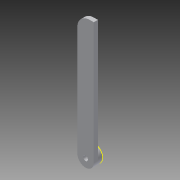
# Autodesk Inventor part: PinewoodStartArm
Saved by Autodesk Inventor 2013 (Build 170138000, 138)
## iProperties
Created: 2015-05-14
Part Number: PinewoodStartArm
Material: Generic
Document SubType Name: Modeling
Designer: joshgunnar
Density: 1 g/cm^3
Author: joshgunnar
Autodesk Inventor part; units mm, degrees
ref_plane "YZ Plane" through (0, 0, 0) normal (1, 0, 0) x (0, 1, 0)
ref_plane "XZ Plane" through (0, 0, 0) normal (0, 1, 0) x (-1, 0, 0)
ref_plane "XY Plane" through (0, 0, 0) normal (0, 0, 1) x (1, 0, 0)
sketch "Sketch1" plane through (0, 0, 0) normal (0, 0, 1) x (1, 0, 0)
  circle A0 centre (0, 0) radius 6
  line L0 (-6, 0) -> (6, 0)
  line L1 (6, 0) -> (6, 88.9)
  line L2 (6, 88.9) -> (-6, 88.9)
  line L3 (-6, 88.9) -> (-6, 0)
  dimension "d0" = 12
  dimension "d1" = 88.9
  constraints: 8 end point, 2 parallel, 1 coincident, 1 horizontal, 1 horizontal alignment, 1 perpendicular, 2 other
  measures "d1" distance of L1.end L0.end
extrude "Extrusion1" add sketch "Sketch1" along normal blind 3
sketch "Sketch2" plane through (0, 0, 0) normal (0, 0, -1) x (-1, 0, 0)
  arc A0 (-6, 0) -> (6, 0) centre (0, 0) ccw projected
  circle A1 centre (0, 0) radius 6
  dimension "d4" = 12
  constraints: 1 centre point, 1 coincident
  measures "d4" diameter of A1
extrude "Extrusion2" add sketch "Sketch2" along normal blind 3.5
sketch "Sketch3" plane through (0, 0, -3.5) normal (0, 0, -1) x (-1, 0, 0)
  circle A0 centre (0, 0) radius 6 projected
  circle A1 centre (0, 0) radius 2.9
  dimension "d7" = 5.8
  constraints: 1 centre point, 1 coincident
  measures "d7" diameter of A1
extrude "Extrusion3" cut sketch "Sketch3" against normal blind 3.5 contours A1
sketch "Sketch5" plane through (0, 0, 0) normal (0, 0, -1) x (-1, 0, 0)
  line L0 (-2.998, 23.4218) -> (-2.998, 33.3533) construction
  line L1 (-2.998, 33.3533) -> (56.8825, 33.3533) construction
  line L2 (56.8825, 33.3533) -> (56.8825, 23.4218) construction
  line L3 (56.8825, 23.4218) -> (-2.998, 23.4218) construction
  spline S0 degree 2 poles (3.3195, 27.1936) (3.3195, 26.1456) (3.0476, 24.5538) (2.8499, 23.8717) knots 0 0 0 1 2 2 2
  line L4 (2.8499, 23.8717) -> (1.3966, 23.8717)
  line L5 (1.3966, 23.8717) -> (1.3966, 24.0793)
  spline S1 degree 2 poles (1.3966, 24.0793) (1.7871, 24.7664) (2.2073, 26.4273) (2.2073, 27.2084) knots 0 0 0 1 2 2 2
  spline S2 degree 2 poles (2.2073, 27.2084) (2.2073, 27.4012) (2.148, 28.0487) (2.0886, 28.2415) knots 0 0 0 1 2 2 2
  spline S3 degree 2 poles (2.0886, 28.2415) (2.0194, 28.4838) (1.7673, 28.8149) (1.5647, 28.8149) knots 0 0 0 1 2 2 2
  spline S4 degree 2 poles (1.5647, 28.8149) (1.3323, 28.8149) (1.0456, 28.2761) (0.9814, 27.9004) knots 0 0 0 1 2 2 2
  spline S5 degree 2 poles (0.9814, 27.9004) (0.8973, 27.4308) (0.754, 26.373) (0.6452, 25.9083) knots 0 0 0 1 2 2 2
  spline S6 degree 2 poles (0.6452, 25.9083) (0.398, 24.8455) (-0.4473, 23.9261) (-1.08, 23.9261) knots 0 0 0 1 2 2 2
  spline S7 degree 2 poles (-1.08, 23.9261) (-1.9352, 23.9261) (-2.998, 26.1011) (-2.998, 27.7274) knots 0 0 0 1 2 2 2
  spline S8 degree 2 poles (-2.998, 27.7274) (-2.998, 28.548) (-2.7755, 30.1645) (-2.5877, 30.8021) knots 0 0 0 1 2 2 2
  line L6 (-2.5877, 30.8021) -> (-1.1937, 30.8021)
  line L7 (-1.1937, 30.8021) -> (-1.1937, 30.5995)
  spline S9 degree 2 poles (-1.1937, 30.5995) (-1.4853, 30.0903) (-1.8857, 28.6222) (-1.8857, 27.8461) knots 0 0 0 1 2 2 2
  spline S10 degree 2 poles (-1.8857, 27.8461) (-1.8857, 27.5445) (-1.8264, 27.065) (-1.7473, 26.803) knots 0 0 0 1 2 2 2
  spline S11 degree 2 poles (-1.7473, 26.803) (-1.6831, 26.5855) (-1.426, 26.2741) (-1.2678, 26.2741) knots 0 0 0 1 2 2 2
  spline S12 degree 2 poles (-1.2678, 26.2741) (-1.0306, 26.2741) (-0.7587, 26.7734) (-0.6499, 27.4852) knots 0 0 0 1 2 2 2
  spline S13 degree 2 poles (-0.6499, 27.4852) (-0.5807, 27.9449) (-0.4473, 28.8001) (-0.3336, 29.2846) knots 0 0 0 1 2 2 2
  spline S14 degree 2 poles (-0.3336, 29.2846) (-0.1012, 30.2337) (0.6699, 31.163) (1.3027, 31.163) knots 0 0 0 1 2 2 2
  spline S15 degree 2 poles (1.3027, 31.163) (2.2122, 31.163) (3.3195, 29.0176) (3.3195, 27.1936) knots 0 0 0 1 2 2 2
  line L8 (3.2108, 34.0894) -> (-1.7276, 34.0894)
  line L9 (-1.7276, 34.0894) -> (-1.7276, 31.3855)
  line L10 (-1.7276, 31.3855) -> (-2.8892, 31.3855)
  line L11 (-2.8892, 31.3855) -> (-2.8892, 39.092)
  line L12 (-2.8892, 39.092) -> (-1.7276, 39.092)
  line L13 (-1.7276, 39.092) -> (-1.7276, 36.388)
  line L14 (-1.7276, 36.388) -> (3.2108, 36.388)
  line L15 (3.2108, 36.388) -> (3.2108, 34.0894)
  line L16 (3.2108, 39.0525) -> (-2.8892, 42.142)
  line L17 (-2.8892, 42.142) -> (-2.8892, 44.6433)
  line L18 (-2.8892, 44.6433) -> (3.2108, 47.7329)
  line L19 (3.2108, 47.7329) -> (3.2108, 45.365)
  line L20 (3.2108, 45.365) -> (1.9651, 44.7966)
  line L21 (1.9651, 44.7966) -> (1.9651, 41.9295)
  line L22 (1.9651, 41.9295) -> (3.2108, 41.356)
  line L23 (3.2108, 41.356) -> (3.2108, 39.0525)
  line L24 (0.8578, 44.2923) -> (-1.1492, 43.363)
  line L25 (-1.1492, 43.363) -> (0.8578, 42.4337)
  line L26 (0.8578, 42.4337) -> (0.8578, 44.2923)
  line L27 (3.2108, 57.1053) -> (3.2108, 54.3074)
  line L28 (3.2108, 54.3074) -> (0.9715, 51.7567)
  line L29 (0.9715, 51.7567) -> (0.9715, 50.9262)
  line L30 (0.9715, 50.9262) -> (3.2108, 50.9262)
  line L31 (3.2108, 50.9262) -> (3.2108, 48.6424)
  line L32 (3.2108, 48.6424) -> (-2.8892, 48.6424)
  line L33 (-2.8892, 48.6424) -> (-2.8892, 52.3252)
  spline S16 degree 2 poles (-2.8892, 52.3252) (-2.8892, 53.0864) (-2.7607, 54.2184) (-2.563, 54.6979) knots 0 0 0 1 2 2 2
  spline S17 degree 2 poles (-2.563, 54.6979) (-2.3554, 55.1873) (-1.7078, 55.7657) (-1.2135, 55.7657) knots 0 0 0 1 2 2 2
  spline S18 degree 2 poles (-1.2135, 55.7657) (-0.5165, 55.7657) (0.3585, 54.8215) (0.6155, 54.0256) knots 0 0 0 1 2 2 2
  line L34 (0.6155, 54.0256) -> (3.2108, 57.1053)
  spline S19 degree 2 poles (-1.0207, 53.4077) (-1.253, 53.4077) (-1.5842, 53.1408) (-1.6732, 52.8343) knots 0 0 0 1 2 2 2
  spline S20 degree 2 poles (-1.6732, 52.8343) (-1.7325, 52.6218) (-1.7671, 52.0879) (-1.7671, 51.6974) knots 0 0 0 1 2 2 2
  line L35 (-1.7671, 51.6974) -> (-1.7671, 50.9262)
  line L36 (-1.7671, 50.9262) -> (-0.1259, 50.9262)
  line L37 (-0.1259, 50.9262) -> (-0.1259, 51.5837)
  spline S21 degree 2 poles (-0.1259, 51.5837) (-0.1259, 52.0632) (-0.205, 52.7355) (-0.3286, 52.9727) knots 0 0 0 1 2 2 2
  spline S22 degree 2 poles (-0.3286, 52.9727) (-0.4473, 53.1902) (-0.7636, 53.4077) (-1.0207, 53.4077) knots 0 0 0 1 2 2 2
  line L38 (3.2108, 59.5374) -> (-1.7276, 59.5374)
  line L39 (-1.7276, 59.5374) -> (-1.7276, 56.8334)
  line L40 (-1.7276, 56.8334) -> (-2.8892, 56.8334)
  line L41 (-2.8892, 56.8334) -> (-2.8892, 64.54)
  line L42 (-2.8892, 64.54) -> (-1.7276, 64.54)
  line L43 (-1.7276, 64.54) -> (-1.7276, 61.836)
  line L44 (-1.7276, 61.836) -> (3.2108, 61.836)
  line L45 (3.2108, 61.836) -> (3.2108, 59.5374)
  constraints: 2 other
extrude "Extrusion5" add sketch "Sketch5" along normal blind 1.5
sketch "Sketch6" plane through (0, 0, 3) normal (0, 0, 1) x (1, 0, 0)
  arc A0 (-6, 0) -> (6, 0) centre (0, 0) ccw projected
  circle A1 centre (0, 0) radius 1.75
  dimension "d18" = 3.5
  constraints: 1 centre point, 1 coincident
  measures "d18" diameter of A1
extrude "Extrusion6" cut sketch "Sketch6" against normal through all
fillet "Fillet2" radius 9 1 edges at (-6, 88.9, 1.5)
sketch "Sketch7" plane through (0, 0, -3.5) normal (0, 0, -1) x (-1, 0, 0)
  circle A0 centre (0, 0) radius 2.9 projected
  circle A1 centre (0, 0) radius 6 projected
sketch "Sketch8" plane through (0, 0, -3.5) normal (0, 0, -1) x (-1, 0, 0)
  line L0 (-0.1588, 2.7978) -> (0, 3.6515)
  line L1 (0, 3.6515) -> (0.1599, 2.7385)
  line L2 (0.1599, 2.7385) -> (-0.1588, 2.7978)
  constraints: 6 end point, 1 perpendicular
extrude "Extrusion7" cut sketch "Sketch8" against normal blind 3.5
pattern_circular "Circular Pattern2" count 60 over 360 about axis through (0, 0, -10) along (0, 0, 1) of "Extrusion7"
body "Solid1"
